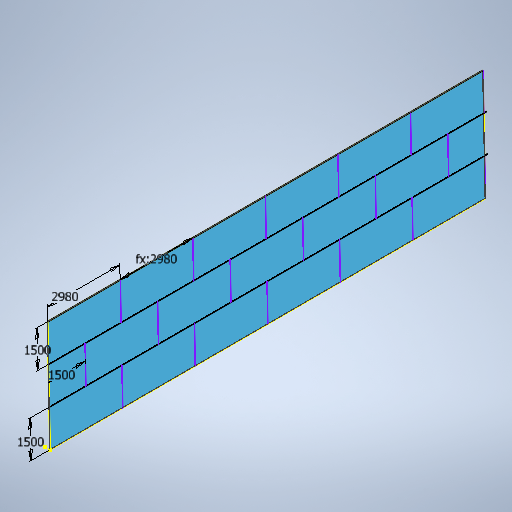
# Autodesk Inventor part: GBK dummy wall 1
Saved by Autodesk Inventor 2026.2 (Build 302298000, 298)
## iProperties
Created: 2026-05-13
Part Number: GBK dummy wall 1
Material: Generic
Document SubType Name: Modeling
Designer: admin
Density: 1 g/cm^3
Appearance: Default
Author: admin
Autodesk Inventor part; units mm, degrees
ref_plane "YZ Plane" through (0, 0, 0) normal (1, 0, 0) x (0, 1, 0)
ref_plane "XZ Plane" through (0, 0, 0) normal (0, 1, 0) x (-1, 0, 0)
ref_plane "XY Plane" through (0, 0, 0) normal (0, 0, 1) x (1, 0, 0)
sketch "Sketch1" plane through (0, 0, 0) normal (0, 0, 1) x (1, 0, 0)
  line L0 (200, 0) -> (190, 0)
  line L1 (190, 0) -> (90.0049, 4499.7779)
  line L2 (90.0049, 4499.7779) -> (100, 4500)
  line L3 (100, 4500) -> (200, 0)
  line L4 (0, 4500) -> (0, 0)
  dimension "d0" = 10
  dimension "d2" = 4500
  dimension "d5" = 100
  dimension "d17" = 200
  constraints: 10 end point, 2 perpendicular, 1 horizontal, 1 horizontal alignment, 1 point on line, 1 vertical
  measures "d0" distance of L0.start L0.end
  measures "d2" distance from line of L0 L2.end
  measures "d5" distance of L2.end L4.start
  measures "d17" distance of L4.end L0.start
extrude "Extrusion1" add sketch "Sketch1" against normal blind 17880
sketch "Sketch2" plane through (0, 0, 0) normal (1, 0, 0) x (0, 1, 0)
  point P0 (0, 0)
sketch "Sketch3" plane through (200, 0, 0) normal (0.9998, 0.0222, 0) x (0, 0, -1)
  line L0 (0, 0) -> (0, 4501.111) projected
  line L1 (0, 0) -> (17880, 0) projected
  line L2 (17880, 4501.111) -> (17880, 0) projected
  line L3 (0, 4501.111) -> (17880, 4501.111)
  line L4 (0, 1500) -> (18000, 1500)
  line L5 (0, 3001.111) -> (18000, 3001.111)
  line L6 (1500, 3001.111) -> (1500, 1500)
  line L7 (0, 4501.111) -> (17880, 4501.111) projected
  line L8 (2980, 4501.111) -> (2980, 3001.111)
  line L9 (2980, 1500) -> (2980, 0)
  line L10 (5960, 4501.111) -> (5960, 3001.111)
  line L11 (4480, 3001.111) -> (4480, 1500)
  line L12 (5960, 1500) -> (5960, 0)
  line L13 (8940, 4501.111) -> (8940, 3001.111)
  line L14 (7460, 3001.111) -> (7460, 1500)
  line L15 (8940, 1500) -> (8940, 0)
  line L16 (11920, 4501.111) -> (11920, 3001.111)
  line L17 (10440, 3001.111) -> (10440, 1500)
  line L18 (11920, 1500) -> (11920, 0)
  line L19 (14900, 4501.111) -> (14900, 3001.111)
  line L20 (13420, 3001.111) -> (13420, 1500)
  line L21 (14900, 1500) -> (14900, 0)
  line L22 (17880, 4501.111) -> (17880, 3001.111)
  line L23 (16400, 3001.111) -> (16400, 1500)
  line L24 (17880, 1500) -> (17880, 0)
  point P0 (0, 4.4433)
  dimension "d6" = 2980
  dimension "d7" = 1500
  dimension "d8" = 1500
  dimension "d9" = 1500
  dimension "d12" = 2980
  constraints: 42 end point, 17 point on line, 3 horizontal, 2 perpendicular, 46 other
  measures "d6" distance between parallel lines of L0 L8
  measures "d7" distance between parallel lines of L0 L6
  measures "d8" distance between parallel lines of L5 L3
  measures "d9" distance between parallel lines of L1 L4
  measures "d12" distance of L8.start L10.start
equation "\"d12\" = d6"
body "Solid1"
